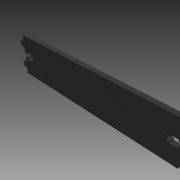
# Autodesk Inventor part: front_panel_2004_front
Saved by Autodesk Inventor 2014 (Build 180170000, 170)
## iProperties
Created: 2014-01-11
Part Number: front_panel_2004_front
Material: Generic
Document SubType Name: Modeling
Designer: buben
Density: 1 g/cm^3
Appearance: Anodized - Dark Gray
Author: buben
Autodesk Inventor part; units mm, degrees
ref_plane "YZ Plane" through (0, 0, 0) normal (1, 0, 0) x (0, 1, 0)
ref_plane "XZ Plane" through (0, 0, 0) normal (0, 1, 0) x (-1, 0, 0)
ref_plane "XY Plane" through (0, 0, 0) normal (0, 0, 1) x (1, 0, 0)
sketch "Sketch1" plane through (0, 0, 0) normal (0, 1, 0) x (-1, 0, 0)
  line L0 (0, 0) -> (220, 0)
  line L1 (220, 0) -> (220, 53.1)
  line L2 (220, 53.1) -> (0, 53.1)
  line L3 (0, 53.1) -> (0, 0)
  dimension "d0" = 53.1
  dimension "d1" = 220
  constraints: 8 end point, 2 parallel, 1 horizontal, 1 perpendicular
  measures "d0" distance of L2.end L0.start
  measures "d1" distance of L1.end L2.end
extrude "Extrusion1" add sketch "Sketch1" along normal blind 6
sketch "Sketch2" plane through (0, 6, 0) normal (0, 1, 0) x (1, 0, 0)
  line L0 (-220, 0) -> (-220, -53.1) projected
  line L1 (0, -53.1) -> (0, 0) projected
  line L2 (-220, -8.0055) -> (-224, -8.0055)
  line L3 (-226, -10.0055) -> (-226, -14.0055)
  line L4 (-224, -16.0055) -> (-220, -16.0055)
  line L5 (-220, -16.0055) -> (-220, -8.0055)
  line L6 (-220, -37.0945) -> (-224, -37.0945)
  line L7 (-226, -39.0945) -> (-226, -43.0945)
  line L8 (-224, -45.0945) -> (-220, -45.0945)
  line L9 (-220, -45.0945) -> (-220, -37.0945)
  line L10 (0, -8.0055) -> (4, -8.0055)
  line L11 (6, -10.0055) -> (6, -14.0055)
  line L12 (4, -16.0055) -> (0, -16.0055)
  line L13 (0, -16.0055) -> (0, -8.0055)
  line L14 (0, -37.0945) -> (4, -37.0945)
  line L15 (6, -39.0945) -> (6, -43.0945)
  line L16 (4, -45.0945) -> (0, -45.0945)
  line L17 (0, -45.0945) -> (0, -37.0945)
  arc A0 (-224, -8.0055) -> (-226, -10.0055) centre (-224, -10.0055) ccw
  arc A1 (-226, -14.0055) -> (-224, -16.0055) centre (-224, -14.0055) ccw
  arc A2 (-224, -37.0945) -> (-226, -39.0945) centre (-224, -39.0945) ccw
  arc A3 (-226, -43.0945) -> (-224, -45.0945) centre (-224, -43.0945) ccw
  arc A4 (4, -45.0945) -> (6, -43.0945) centre (4, -43.0945) ccw
  arc A5 (6, -39.0945) -> (4, -37.0945) centre (4, -39.0945) ccw
  arc A6 (4, -16.0055) -> (6, -14.0055) centre (4, -14.0055) ccw
  arc A7 (6, -10.0055) -> (4, -8.0055) centre (4, -10.0055) ccw
  line L18 (-222, -16.0055) -> (-222, -37.0945) construction
  point P0 (-222, -26.55)
  point P1 (-220, -26.55)
  dimension "d4" = 2
  dimension "d5" = 8
  dimension "d6" = 8
  dimension "d7" = 6
  dimension "d8" = 6
  dimension "d9" = 21.089
  constraints: 34 end point, 16 point on circle, 16 tangent, 8 centre point, 8 parallel, 7 equal radius, 6 collinear, 4 horizontal, 4 midpoint, 4 perpendicular, 4 point on line, 1 horizontal alignment
  measures "d4" radius of A0
  measures "d5" distance between parallel lines of L4 L2
  measures "d6" distance between parallel lines of L8 L6
  measures "d7" distance between parallel lines of L0 L3
  measures "d8" distance between parallel lines of L1 L11
  measures "d9" distance of L18.start L18.end
extrude "Extrusion2" add sketch "Sketch2" against normal blind 6
sketch "Sketch3" plane through (0, 6, 0) normal (0, 1, 0) x (1, 0, 0)
  line L0 (0, 0) -> (-220, 0) projected
  line L1 (-220, -16.0055) -> (-220, -37.0945) projected
  line L2 (-220, -53.1) -> (0, -53.1) projected
  line L3 (-203.7, -24.3) -> (-203.7, -28.8)
  line L4 (-220, -28.8) -> (-220, -24.3)
  line L5 (-215, -21.8) -> (-207.7, -21.8)
  line L6 (-207.7, -31.3) -> (-215, -31.3)
  line L7 (-220, -24.3) -> (-215, -24.3)
  line L8 (-207.7, -24.3) -> (-203.7, -24.3)
  line L9 (-203.7, -28.8) -> (-207.7, -28.8)
  line L10 (-215, -28.8) -> (-220, -28.8)
  line L11 (-207.7, -21.8) -> (-207.7, -24.3)
  line L12 (-207.7, -28.8) -> (-207.7, -31.3)
  line L13 (-215, -31.3) -> (-215, -28.8)
  line L14 (-215, -24.3) -> (-215, -21.8)
  line L15 (-110, 0) -> (-110, -53.1) construction
  line L16 (-16.3, -24.3) -> (-16.3, -28.8)
  line L17 (0, -28.8) -> (0, -24.3)
  line L18 (-5, -21.8) -> (-12.3, -21.8)
  line L19 (-12.3, -31.3) -> (-5, -31.3)
  line L20 (0, -24.3) -> (-5, -24.3)
  line L21 (-12.3, -24.3) -> (-16.3, -24.3)
  line L22 (-16.3, -28.8) -> (-12.3, -28.8)
  line L23 (-5, -28.8) -> (0, -28.8)
  line L24 (-12.3, -21.8) -> (-12.3, -24.3)
  line L25 (-12.3, -28.8) -> (-12.3, -31.3)
  line L26 (-5, -31.3) -> (-5, -28.8)
  line L27 (-5, -24.3) -> (-5, -21.8)
  point P0 (-203.7, -26.55)
  point P1 (-220, -26.55)
  point P2 (-16.3, -26.55)
  point P3 (0, -26.55)
  dimension "d12" = 4.5
  dimension "d13" = 2.5
  dimension "d14" = 2.5
  dimension "d15" = 5
  dimension "d16" = 4
  dimension "d17" = 7.3
  constraints: 50 end point, 14 symmetric about line, 10 parallel, 5 collinear, 4 midpoint, 4 perpendicular, 3 horizontal, 1 horizontal alignment
  measures "d12" distance of L3.start L3.end
  measures "d13" distance of L5.end L8.start
  measures "d14" distance of L9.end L6.start
  measures "d15" distance of L10.start L4.start
  measures "d16" distance of L3.end L9.end
  measures "d17" distance of L6.start L6.end
extrude "Extrusion3" cut sketch "Sketch3" against normal blind 6
body "Solid1"
